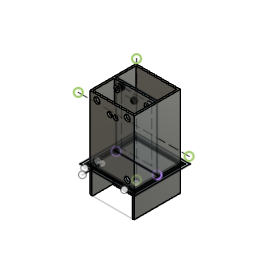
EMI_BOX v7 (Autodesk Fusion 360 design; units mm, degrees)
Autodesk Fusion 360 part; units mm, degrees
note: some values were not read from the file. Set by a fixed rule: which face or edge a step refers to.
sketch "Sketch1" plane through (0, 0, 0) normal (0, 0, 1) x (1, 0, 0)
  line L0 (0, 50) -> (0, -40) construction
  line L1 (-50, 0) -> (45, 0) construction
  line L2 (-17.5, 27.5) -> (17.5, 27.5)
  line L3 (17.5, 27.5) -> (17.5, -27.5)
  line L4 (17.5, -27.5) -> (-17.5, -27.5)
  line L5 (-17.5, -27.5) -> (-17.5, 27.5)
  line L6 (-13, 23) -> (13, 23) construction
  line L7 (13, 23) -> (13, -23) construction
  line L8 (13, -23) -> (-13, -23) construction
  line L9 (-13, -23) -> (-13, 23) construction
  circle A0 centre (-13, 23) radius 2.5
  circle A1 centre (-13, 23) radius 1
  line L10 (-13, 23) -> (-2, 23) construction
  line L11 (-2, 23) -> (-2, 18) construction
  line L12 (-2, 18) -> (-13, 18) construction
  line L13 (-13, 18) -> (-13, 23) construction
  circle A2 centre (-2, 18) radius 2
  dimension "d1" = 35
  dimension "d2" = 55
  dimension "d3" = 17.5
  dimension "d4" = 27.5
  dimension "d5" = 26
  dimension "d6" = 46
  dimension "d7" = 13
  dimension "d8" = 23
  dimension "d9" = 5
  dimension "d10" = 2
  dimension "d63" = 11
  dimension "d64" = 5
  dimension "d65" = 4
  constraint vertical L0
  constraint horizontal L1
  constraint horizontal L2
  constraint vertical L3
  constraint horizontal L4
  constraint vertical L5
  constraint horizontal L6
  constraint vertical L7
  constraint horizontal L8
  constraint vertical L9
  constraint coincident L6.start L9.end
  constraint horizontal L10
  constraint vertical L11
  constraint horizontal L12
  constraint vertical L13
  constraint coincident L11.end L12.start
  measures "d1" distance of L2.start L2.end
  measures "d2" distance of L2.start L4.end
  measures "d3" distance of L0 L3
  measures "d4" distance of L1 L4
  measures "d5" distance of L6.start L6.end
  measures "d6" distance of L6.start L8.end
  measures "d7" distance of L0 L7
  measures "d8" distance of L1 L8
  measures "d9" diameter of A0
  measures "d10" diameter of A1
  measures "d63" distance of L6.start L10.end
  measures "d64" distance of L6.start L12.end
  measures "d65" diameter of A2
extrude "Extrude1" add sketch "Sketch1" along normal blind 4 contours A0 makes body 1
pattern_linear "R-Pattern1" count 2 spacing 46 along (0, -1, 0) count 2 spacing 26 along (1, 0, 0) of bodies 1 makes body 2 at (-10.5031, -23.1246, 2.6667) makes body 3 at (15.4969, 22.8754, 2.6667) makes body 4 at (15.4969, -23.1246, 2.6667)
extrude "Extrude2" add sketch "Sketch1" along normal blind 1.5 separate body contours L2 L3 L4 L5 | A2 makes body 5
sketch "Sketch2" plane through (0, -27.5, 0) normal (0, -1, 0) x (1, 0, 0)
  line L0 (-17.5, 0) -> (17.5, 0)
  line L1 (17.5, 0) -> (17.5, 1.5)
  line L2 (17.5, 1.5) -> (-17.5, 1.5)
  line L3 (-17.5, 1.5) -> (-17.5, 0)
  line L4 (-17.5, 0) -> (17.5, 0)
  line L5 (17.5, 0) -> (17.5, 19.5)
  line L6 (17.5, 19.5) -> (-17.5, 19.5)
  line L7 (-17.5, 19.5) -> (-17.5, 0)
  line L8 (-19, 21) -> (19, 21)
  line L9 (19, 21) -> (19, 0)
  line L10 (19, 0) -> (-19, 0)
  line L11 (-19, 0) -> (-19, 21)
  line L12 (17.5, 0) -> (-17.5, 0)
  line L13 (-17.5, 0) -> (17.5, 0)
  line L14 (17.5, 0) -> (17.5, -17)
  line L15 (17.5, -17) -> (-17.5, -17)
  line L16 (-17.5, -17) -> (-17.5, 0)
  line L17 (-19, 0) -> (19, 0)
  line L18 (19, 0) -> (19, -18.5)
  line L19 (19, -18.5) -> (-19, -18.5)
  line L20 (-19, -18.5) -> (-19, 0)
  line L21 (-20.5, -19.25) -> (20.5, -19.25)
  line L22 (20.5, -19.25) -> (20.5, 21.75)
  line L23 (20.5, 21.75) -> (-20.5, 21.75)
  line L24 (-20.5, 21.75) -> (-20.5, -19.25)
  line L25 (-19, -17.75) -> (19, -17.75)
  line L26 (19, -17.75) -> (19, 20.25)
  line L27 (19, 20.25) -> (-19, 20.25)
  line L28 (-19, 20.25) -> (-19, -17.75)
  line L29 (-21.5, -20.25) -> (21.5, -20.25)
  line L30 (21.5, -20.25) -> (21.5, 22.75)
  line L31 (21.5, 22.75) -> (-21.5, 22.75)
  line L32 (-21.5, 22.75) -> (-21.5, -20.25)
  line L33 (-18.5, 15) -> (-18.5, 26)
  line L34 (14.5, 15) -> (14.5, 25)
  line L35 (-23.5, -22.25) -> (23.5, -22.25)
  line L36 (23.5, -22.25) -> (23.5, 24.75)
  line L37 (23.5, 24.75) -> (-23.5, 24.75)
  line L38 (-23.5, 24.75) -> (-23.5, -22.25)
  line L39 (-14.5, 15) -> (-14.5, 32)
  dimension "d19" = 35
  dimension "d20" = 19.5
  dimension "d22" = 1.5
  dimension "d23" = 1.5
  dimension "d24" = 1.5
  dimension "d25" = 17
  dimension "d83" = 1.5
  dimension "d86" = 3
  dimension "d88" = 2.25
  dimension "d90" = 2.25
  dimension "d91" = 1.5
  dimension "d92" = 1.5
  dimension "d93" = 1.5
  dimension "d94" = 1.5
  dimension "d100" = 1
  dimension "d101" = 1
  dimension "d102" = 1
  dimension "d103" = 1
  dimension "d104" = 2
  dimension "d105" = 6
  dimension "d112" = 2
  dimension "d113" = 2
  dimension "d114" = 2
  dimension "d115" = 2
  dimension "d118" = 3
  dimension "d119" = 3
  constraint horizontal L4
  constraint vertical L5
  constraint horizontal L6
  constraint vertical L7
  constraint coincident L0.start L3.end
  constraint horizontal L8
  constraint vertical L9
  constraint horizontal L10
  constraint vertical L11
  constraint collinear L10 L12
  constraint horizontal L13
  constraint vertical L14
  constraint horizontal L15
  constraint vertical L16
  constraint horizontal L17
  constraint vertical L18
  constraint horizontal L19
  constraint vertical L20
  constraint horizontal L21
  constraint vertical L22
  constraint horizontal L23
  constraint vertical L24
  constraint collinear L5 L14
  constraint collinear L9 L18
  constraint horizontal L25
  constraint vertical L26
  constraint horizontal L27
  constraint vertical L28
  constraint horizontal L29
  constraint vertical L30
  constraint horizontal L31
  constraint vertical L32
  constraint perpendicular L6 L33
  constraint perpendicular L31 L34
  constraint horizontal L35
  constraint vertical L36
  constraint horizontal L37
  constraint vertical L38
  constraint perpendicular L37 L39
  measures "d19" distance of L0.start L0.end
  measures "d20" distance of L0.start L6.end
  measures "d22" distance of L7 L11
  measures "d23" distance of L6 L8
  measures "d24" distance of L5 L9
  measures "d25" distance of L0.start L15.end
  measures "d83" distance of L15 L19
  measures "d86" distance of L14 L22
  measures "d88" distance of L15 L21
  measures "d90" distance of L6 L23
  measures "d91" distance of L24 L28
  measures "d92" distance of L22 L26
  measures "d93" distance of L21 L25
  measures "d94" distance of L23 L27
  measures "d100" distance of L21 L29
  measures "d101" distance of L24 L32
  measures "d102" distance of L22 L30
  measures "d103" distance of L23 L31
  measures "d104" distance of L24 L33
  measures "d105" distance of L22 L34
  measures "d112" distance of L32 L38
  measures "d113" distance of L29 L35
  measures "d114" distance of L31 L37
  measures "d115" distance of L30 L36
  measures "d118" distance of L7 L39
  measures "d119" distance of L16 L24
extrude "Extrude3" add sketch "Sketch2" against normal blind 55 contours L3 L6 L7 L10 L11 L17 L27 L28 L39 | L10 L14 L15 L16 L17 L18 L20 L25 L26 L28 | L1 L5 L6 L9 L10 L17 L26 L27 L34 | L8 L11 L27 L33 | L18 L19 L20 L25 | L8 L9 L27 L34 | L6 L27 L34 L39 | L8 L27 L33 L39 | L8 L27 L34 L39 bodies 5
extrude "Extrude4" add sketch "Sketch2" along normal blind 1.5 separate body contours L0 L4 L10 L12 L13 L14 L15 L16 L17 makes body 6
extrude "Extrude5" add sketch "Sketch2" along normal blind 21.5 contours L10 L14 L15 L16 L17 L18 L20 L25 L26 L28 | L18 L19 L20 L25 bodies 5 6
sketch "Sketch3" plane through (0, -49, 0) normal (0, -1, 0) x (1, 0, 0)
  line L0 (17.5, 0) -> (17.5, -17)
  line L1 (17.5, -17) -> (-17.5, -17)
  line L2 (-17.5, -17) -> (-17.5, 0)
  line L3 (-17.5, 0) -> (-19, 0)
  line L4 (-19, 0) -> (-19, -18.5)
  line L5 (-19, -18.5) -> (19, -18.5)
  line L6 (19, -18.5) -> (19, 0)
  line L7 (19, 0) -> (17.5, 0)
  line L8 (-19, 0) -> (19, 0)
  line L9 (19, 0) -> (19, -18.5)
  line L10 (19, -18.5) -> (-19, -18.5)
  line L11 (-19, -18.5) -> (-19, 0)
  line L12 (-46.8165, -8.5) -> (11.8165, -8.5) construction
  line L13 (-17.5, -17) -> (-17.5, 0) construction
  line L14 (0, -10.2369) -> (0, -23.7631) construction
  line L15 (17.5, -17) -> (-17.5, -17) construction
  line L16 (-10.5, -1.75) -> (10.5, -1.75)
  line L17 (10.5, -1.75) -> (10.5, -15.25)
  line L18 (10.5, -15.25) -> (-10.5, -15.25)
  line L19 (-10.5, -15.25) -> (-10.5, -1.75)
  dimension "d32" = 21
  dimension "d33" = 13.5
  dimension "d34" = 10.5
  dimension "d35" = 6.75
  constraint horizontal L8
  constraint vertical L9
  constraint horizontal L10
  constraint vertical L11
  constraint coincident L5.end L6.start
  constraint coincident L3.end L4.start
  constraint horizontal L12
  constraint midpoint L12 L13
  constraint perpendicular L12 L14
  constraint midpoint L14 L15
  constraint horizontal L16
  constraint vertical L17
  constraint horizontal L18
  constraint vertical L19
  measures "d32" distance of L16.start L16.end
  measures "d33" distance of L16.start L18.end
  measures "d34" distance of L14 L19
  measures "d35" distance of L12 L16
extrude "Extrude6" add sketch "Sketch3" along normal blind 1.5 separate body makes body 7
sketch "Sketch4" plane through (0, 0, 4) normal (0, 0, 1) x (1, 0, 0)
  circle A0 centre (-13, 23) radius 1
  circle A1 centre (-13, 23) radius 2.5
extrude "Extrude8" add sketch "Sketch4" along normal blind 20 separate body contours A0 | A1 makes body 8
pattern_linear "R-Pattern2" count 2 spacing 46 along (0, -1, 0) count 2 spacing 26 along (1, 0, 0) of bodies 8 makes body 9 at (-10.5031, -23.1246, 17.3333) makes body 10 at (15.4969, 22.8754, 17.3333) makes body 11 at (15.4969, -23.1246, 17.3333)
combine "Combine1" operation cut target body 5 tool bodies 11 10 9 8
sketch "Sketch5" plane through (0, -27.5, 0) normal (0, -1, 0) x (1, 0, 0)
  line L0 (-19, 0) -> (-17.5, 0)
  line L1 (-17.5, 0) -> (-17.5, 21)
  line L2 (-17.5, 21) -> (-19, 21)
  line L3 (-19, 21) -> (-19, 0)
  line L4 (-19, 21) -> (19, 21)
  line L5 (17.5, 0) -> (19, 0)
  line L6 (19, 0) -> (19, 21)
  line L7 (19, 21) -> (17.5, 21)
  line L8 (17.5, 21) -> (17.5, 0)
  point P0 (-19, 0)
  point P1 (17.5, 0)
  constraint horizontal L0
  constraint vertical L1
  constraint horizontal L2
  constraint vertical L3
  constraint coincident L1.end L4
  constraint coincident P0 L0.start
  constraint horizontal L5
  constraint vertical L6
  constraint horizontal L7
  constraint vertical L8
  constraint coincident L4.end L6.end
  constraint coincident P1 L5.start
extrude "Extrude9" add sketch "Sketch5" along normal blind 23 bodies 7 5
sketch "Sketch6" plane through (0, 0, 0) normal (0, 0, 1) x (1, 0, 0)
  line L0 (-17.5, -27.5) -> (-17.5, -29)
  line L1 (-17.5, -29) -> (17.5, -29)
  line L2 (17.5, -29) -> (17.5, -27.5)
  line L3 (17.5, -27.5) -> (-17.5, -27.5)
extrude "Extrude10" add sketch "Sketch6" along normal blind 1.5 bodies 7
sketch "Sketch7" plane through (0, -29, 0) normal (0, -1, 0) x (1, 0, 0)
  line L0 (-17.5, -17) -> (17.5, -17)
  line L1 (17.5, -17) -> (17.5, 1.5)
  line L2 (17.5, 1.5) -> (-17.5, 1.5)
  line L3 (-17.5, 1.5) -> (-17.5, -17)
  circle A0 centre (-15, -7) radius 2
  dimension "d50" = 4
  measures "d50" diameter of A0
extrude "Extrude11" cut sketch "Sketch7" against normal blind 3 contours A0 bodies 7
sketch "Sketch8" plane through (0, 0, 0) normal (0, 0, 1) x (1, 0, 0)
  line L0 (-17.5, -49) -> (-17.5, -50.5)
  line L1 (-17.5, -50.5) -> (17.5, -50.5)
  line L2 (17.5, -50.5) -> (17.5, -49)
  line L3 (17.5, -49) -> (-17.5, -49)
extrude "Extrude12" add sketch "Sketch8" along normal blind 3 bodies 7
extrude "Extrude13" add sketch "Sketch2" along normal blind 1.5 contours L3 L6 L7 L10 L11 L17 L27 L28 L39 | L1 L5 L6 L9 L10 L17 L26 L27 L34 | L8 L11 L27 L33 | L8 L9 L27 L34 | L6 L27 L34 L39 | L8 L27 L33 L39 | L8 L27 L34 L39 bodies 7
combine "Combine2" operation add target body 7 tool bodies 4 3 2 1
extrude "Extrude14" add 1 faces at (-13.5412, -23.1083, 1.5) along direction (0, 0, -1) blind 1.5 separate body on bodies 7 makes body 12
pattern_linear "R-Pattern3" count 2 spacing 46 along (0, 1, 0) count 2 spacing 26 along (1, 0, 0) of bodies 12 makes body 13 at (-12.0012, 23.0498, 0.5) makes body 14 at (13.9988, -22.9502, 0.5) makes body 15 at (13.9988, 23.0498, 0.5)
combine "Combine3" operation cut target body 7 tool bodies 12 13 14 15
extrude "Extrude15" add sketch "Sketch1" along normal blind 20 separate body contours A2 makes body 16
pattern_linear "R-Pattern4" count 2 spacing 5 along (1, 0, 0) of bodies 16 makes body 17
move_body "Move1" bodies 16 17 to x (1, 0, 0) y (0, 1, 0) z (0, 0, 1) at (0, 0, 5)
combine "Combine4" operation cut target body 7 tool bodies 16 17
fillet "Fillet1" radius 1 2 edges at (-18.25, -50.5, 21) (18.25, -50.5, 21) on bodies 7
fillet "Fillet1" radius 1 1 edges at (0, -50.5, -18.5) on bodies 7
fillet "Fillet1" radius 1 2 edges at (19, -50.5, 1.25) (-19, -50.5, 1.25) on bodies 7
extrude "Extrude23" add sketch "Sketch2" along normal blind 10 separate body contours L8 L9 L11 L18 L19 L20 L21 L22 L23 L24 L26 L28 L33 L34 | L8 L11 L27 L33 | L18 L19 L20 L25 | L8 L9 L27 L34 makes body 18
extrude "Extrude24" add sketch "Sketch2" against normal blind 3 contours L8 L9 L11 L18 L19 L20 L21 L22 L23 L24 L26 L28 L33 L34 | L8 L11 L27 L33 | L18 L19 L20 L25 | L8 L9 L27 L34 bodies 18
extrude "Extrude25" add sketch "Sketch2" against normal blind 3 contours L21 L22 L23 L24 L29 L30 L31 L32 L33 L34 bodies 18
extrude "Extrude26" add sketch "Sketch2" against normal blind 20 contours L31 L33 L37 L39 | L29 L30 L31 L32 L33 L34 L35 L36 L37 L38 | L31 L34 L37 L39 bodies 18
extrude "Extrude27" cut sketch "Sketch2" against normal blind 15 contours L31 L33 L37 L39 | L31 L34 L37 L39 bodies 18
hidden bodies 18
equation "d3 = d1 / 2"
equation "d4 = d2 / 2"
equation "d7 = d5 / 2"
equation "d8 = d6 / 2"
equation "e = 1.5 mm"
equation "d22 = e"
equation "d23 = e"
equation "d24 = e"
equation "d26 = -d2"
equation "d28 = e"
equation "d30 = 20 mm + e"
equation "d34 = d32 / 2"
equation "d35 = ( d33 / 2 )"
equation "d36 = e"
equation "d46 = 20 mm + 2 * e"
equation "d48 = e"
equation "d55 = e"
equation "d57 = -e"
equation "d83 = e"
equation "L = 41 mm"
equation "e2 = 2 mm"
equation "d86 = ( L - d19 ) / 2"
equation "d88 = ( L - d20 - d25 ) / 2"
equation "d90 = ( L - d20 - d25 ) / 2"
equation "d91 = e"
equation "d92 = e"
equation "d93 = e"
equation "d94 = e"
equation "LB = 43 mm"
equation "d100 = ( LB - L ) / 2"
equation "d101 = ( LB - L ) / 2"
equation "d102 = ( LB - L ) / 2"
equation "d103 = ( LB - L ) / 2"
equation "d112 = e2"
equation "d113 = e2"
equation "d114 = e2"
equation "d115 = e2"
equation "d119 = ( L - d19 ) / 2"
named bodies: "EMI_BOX", "EMI_Holder"
